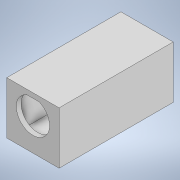
# Autodesk Inventor part: carcasaXeotype_FLEX-SENSOR
Saved by Autodesk Inventor 2020 (Build 240168000, 168)
## iProperties
Created: 2021-04-10
Part Number: carcasaXeotype_FLEX-SENSOR
Material: Generic
Document SubType Name: Modeling
Designer: Vlasciar
Density: 1 g/cm^3
Appearance: Default
Author: Vlasciar
Autodesk Inventor part; units mm, degrees
ref_plane "YZ Plane" through (0, 0, 0) normal (1, 0, 0) x (0, 1, 0)
ref_plane "XZ Plane" through (0, 0, 0) normal (0, 1, 0) x (-1, 0, 0)
ref_plane "XY Plane" through (0, 0, 0) normal (0, 0, 1) x (1, 0, 0)
sketch "Sketch1" plane through (0, 0, 0) normal (0, 1, 0) x (-1, 0, 0)
  line L0 (-5.5, -12) -> (5.5, -12)
  line L1 (5.5, -12) -> (5.5, 12)
  line L2 (5.5, 12) -> (-5.5, 12)
  line L3 (-5.5, 12) -> (-5.5, -12)
  line L4 (-5.5, -12) -> (5.5, 12) construction
  line L5 (5.5, -12) -> (-5.5, 12) construction
  point P0 (0, 0)
  dimension "d0" = 11
  dimension "d1" = 24
  constraints: 12 end point, 2 midpoint, 2 parallel, 1 horizontal, 1 perpendicular
  measures "d0" distance of L1.end L2.end
  measures "d1" distance of L0.end L1.end
extrude "Extrusion1" add sketch "Sketch1" along normal blind 10
shell "Shell1" thickness 1 removed faces 1 at (1.8333, 10, 4)
sketch "Sketch2" plane through (-5.5, 0, 12) normal (0, 0, 1) x (1, 0, 0)
  line L0 (0, 10) -> (11, 10) projected
  circle A0 centre (5.5, 6.75) radius 3.5
  point P0 (5.5, 0)
  point P1 (4.201, 10)
  point P2 (6.799, 10)
  dimension "d5" = 7
  dimension "d6" = 0.25
  constraints: 1 centre point
  measures "d5" diameter of A0
  measures "d6" distance edge to line of A0 L0
extrude "Extrusion2" cut sketch "Sketch2" against normal blind 9 contours L0 A0 picked at (4.7002, 5.9949)
sketch "Sketch3" plane through (0, 10, 0) normal (0, 1, 0) x (1, 0, 0)
  line L0 (1.299, -12) -> (5.5, -12) projected
  line L1 (5.5, -12) -> (5.5, 12) projected
  line L2 (5.5, 12) -> (-5.5, 12) projected
  line L3 (-5.5, 12) -> (-5.5, -12) projected
  line L4 (-5.5, -12) -> (-1.299, -12) projected
  line L5 (-5.5, 12) -> (5.5, 12)
  line L6 (5.5, 12) -> (5.5, -12)
  line L7 (5.5, -12) -> (-5.5, -12)
  line L8 (-5.5, -12) -> (-5.5, 12)
  point P0 (0, 0)
  point P1 (-1.299, -12)
  constraints: 8 end point, 2 parallel, 1 horizontal, 1 perpendicular
extrude "Extrusion3" add sketch "Sketch3" along normal blind 1
sketch "Sketch4" plane through (5.5, 0, -12) normal (0, 0, -1) x (-1, 0, 0)
  line L0 (10, 1) -> (10, 10) projected
  line L1 (1, 1) -> (1, 10) projected
  line L2 (1, 3.25) -> (10, 3.25)
  line L3 (1, 1) -> (10, 1) projected
  line L4 (1, 4.75) -> (10, 4.75)
  line L5 (1.5, 4.75) -> (1.5, 3.25)
  line L6 (9.5, 4.75) -> (9.5, 3.25)
  point P0 (5.5, 0)
  point P1 (10, 3.25)
  dimension "d11" = 2.25
  dimension "d14" = 1.5
  dimension "d15" = 0.5
  dimension "d16" = 0.5
  constraints: 8 end point, 7 point on line, 1 horizontal, 1 parallel, 1 perpendicular
  measures "d11" distance between parallel lines of L3 L2
  measures "d14" distance between parallel lines of L2 L4
  measures "d15" distance between parallel lines of L5 L1
  measures "d16" distance between parallel lines of L0 L6
extrude "Extrusion4" cut sketch "Sketch4" against normal blind 10 contours L2 L6 L4 L0 | L2 L5 L4 L6 | L1 L4 L5 L2
body "Solid1"
